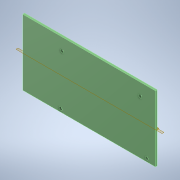
# Autodesk Inventor part: PCB Control Board ADICUP1
Saved by Autodesk Inventor 2021 (Build 250183000, 183)
## iProperties
Created: 2019-11-04
Part Number: PCB Control Board ADICUP1
Material: Generic
Document SubType Name: Modeling
Designer: jgray
Density: 1 g/cm^3
Appearance: Default
Author: jgray
Autodesk Inventor part; units mm, degrees
ref_plane "YZ Plane" through (0, 0, 0) normal (1, 0, 0) x (0, 1, 0)
ref_plane "XZ Plane" through (0, 0, 0) normal (0, 1, 0) x (-1, 0, 0)
ref_plane "XY Plane" through (0, 0, 0) normal (0, 0, 1) x (1, 0, 0)
sketch "Sketch1" plane through (0, 0, 0) normal (0, 0, 1) x (1, 0, 0)
  line L0 (0, 0) -> (127, 0)
  line L1 (127, 0) -> (127, 63)
  line L2 (127, 63) -> (0, 63)
  line L3 (0, 63) -> (0, 0)
  line L4 (13.2018, 51.12) -> (120.6255, 51.12) construction
  line L5 (9.1408, 2.85) -> (116.7218, 2.85) construction
  line L6 (-34.7064, 30.85) -> (160.9804, 30.85)
  point P0 (37.53, 51.12)
  point P1 (112.46, 51.12)
  point P2 (118.81, 2.85)
  point P3 (36.26, 2.85)
  dimension "d0" = 127
  dimension "d1" = 63
  dimension "d21" = 37.53
  dimension "d22" = 36.26
  dimension "d23" = 118.81
  dimension "d24" = 112.46
  dimension "d25" = 30.85
  dimension "d26" = 28
  dimension "d27" = 20.27
  dimension "d28" = 11.88
  dimension "d29" = 2.85
  constraints: 14 end point, 4 horizontal, 4 point on line, 2 parallel, 1 perpendicular
  measures "d0" distance of L2.end L1.end
  measures "d1" distance of L1.end L0.end
  measures "d21" horizontal distance of L2.end point (37.53, 51.12)
  measures "d22" distance from line of L3 point (36.26, 2.85)
  measures "d23" distance from line of L3 point (118.81, 2.85)
  measures "d24" horizontal distance of L2.end point (112.46, 51.12)
  measures "d25" distance between parallel lines of L0 L6
  measures "d26" distance from line of point (118.81, 2.85) L6
  measures "d27" distance from line of point (112.46, 51.12) L6
  measures "d28" distance from line of L2 point (37.53, 51.12)
  measures "d29" distance from line of L0 point (36.26, 2.85)
extrude "Extrusion1" add sketch "Sketch1" along normal blind 1.8
hole "Hole1" at (37.53, 51.12, 0) at (112.46, 51.12, 0) at (118.81, 2.85, 0) at (36.26, 2.85, 0) direction (0, 0, 1) diameter 3.1 end through all
sketch "Sketch2" plane through (0, 0, 1.8) normal (0, 0, 1) x (1, 0, 0)
  line L0 (118.8, 41.95) -> (123.88, 41.95)
  line L1 (123.88, 41.95) -> (123.88, 11.47)
  line L2 (123.88, 11.47) -> (118.8, 11.47)
  line L3 (118.8, 11.47) -> (118.8, 41.95)
  line L4 (127, 0) -> (127, 63) projected
  line L5 (0, 0) -> (127, 0) projected
  dimension "d17" = 5.08
  dimension "d18" = 30.48
  dimension "d19" = 3.12
  dimension "d20" = 11.47
  constraints: 8 end point, 2 parallel, 1 horizontal, 1 perpendicular
  measures "d17" distance of L1.end L2.end
  measures "d18" distance of L0.end L1.end
  measures "d19" distance between parallel lines of L4 L1
  measures "d20" distance between parallel lines of L5 L2
ref_plane "Work Plane1" through (127, 30.85, 0) normal (0, 1, 0) x (1, 0, 0)
body "Solid1"
